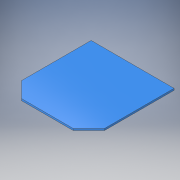
# Autodesk Inventor part: PCB
Saved by Autodesk Inventor 2018 (Build 220112000, 112)
## iProperties
Created: 2019-11-03
Part Number: PCB
Material: Generic
Document SubType Name: Modeling
Designer: jklei
Density: 1 g/cm^3
Appearance: Default
Author: jklei
Autodesk Inventor part; units mm, degrees
ref_plane "YZ Plane" through (0, 0, 0) normal (1, 0, 0) x (0, 1, 0)
ref_plane "XZ Plane" through (0, 0, 0) normal (0, 1, 0) x (-1, 0, 0)
ref_plane "XY Plane" through (0, 0, 0) normal (0, 0, 1) x (1, 0, 0)
sketch "Sketch1" plane through (0, 0, 0) normal (0, 1, 0) x (-1, 0, 0)
  line L0 (0, 0) -> (-73.406, 0)
  line L1 (-73.406, 0) -> (-73.406, -75.438)
  line L2 (-73.406, -75.438) -> (0, -75.438)
  line L3 (0, -75.438) -> (0, 0)
  dimension "d0" = 73.406
  dimension "d1" = 75.438
  constraints: 8 end point, 2 parallel, 1 horizontal, 1 perpendicular
  measures "d0" distance of L2.end L1.end
  measures "d1" distance of L1.end L0.end
extrude "Extrusion1" add sketch "Sketch1" along normal blind 1.5875
chamfer "Chamfer1" distance 13.716 angle 45 2 edges at (0, 0.7937, 0) (73.406, 0.7937, 0)
body "Solid1"
